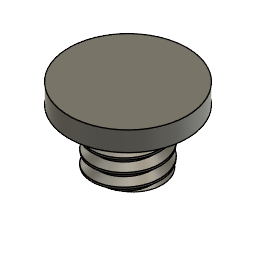
M2.5 x 6mm Phillips Flat Head Screw (Autodesk Fusion 360 design; units mm, degrees)
part number: 2026-08-01-20-11-09-453
Autodesk Fusion 360 part; units mm, degrees
sketch "Sketch1" plane through (0, 0, 0) normal (0, 1, 0) x (1, 0, 0)
  circle A0 centre (0, 0) radius 1.5
  dimension "d1" = 3
  constraint coincident A0.centre origin
  measures "d1" diameter of A0
extrude "Extrude1" add sketch "Sketch1" along normal blind 2
thread "Thread1" "ISO Metric profile 2.5 M2.5x0.45 M2.5x0.45 6g" major diameter 2.43 minor diameter 1.9165 pitch 0.45 angle 60 modelled right hand crest width 0.0648 on face at (1.4981, 1.3333, 0.0748) crest through (1.215, -0.1125, 0)
sketch "Sketch2" plane through (0, 2, 0) normal (0, 1, 0) x (-1, 0, 0)
  spline S0 degree 3 poles (-0.1252, 1.2085) (-0.2764, 1.1771) (-0.4201, 1.117) (-0.6707, 0.9476) (-0.7764, 0.8419) (-0.9369, 0.6004) (-0.9921, 0.4683) (-1.0464, 0.1962) (-1.0473, 0.0593) (-1.0042, -0.1619) (-0.9753, -0.2474) (-0.8966, -0.4057) (-0.8477, -0.4781) (-0.7897, -0.5428) knots 0 0 0 0 0.046326 0.046326 0.090815 0.090815 0.133466 0.133466 0.17428 0.17428 0.201332 0.201332 0.227524 0.227524 0.227524 0.227524
  arc A0 (-0.7897, -0.5428) -> (0.2561, -0.9234) centre (0, 0) ccw
  spline S1 degree 3 poles (0.2561, -0.9234) (0.3815, -0.9055) (0.5022, -0.8627) (0.7262, -0.7312) (0.8263, -0.6416) (0.9913, -0.4249) (1.0527, -0.2985) (1.1264, -0.0233) (1.1356, 0.1233) (1.1038, 0.3714) (1.0763, 0.4727) (0.9942, 0.6681) (0.9393, 0.7609) (0.8727, 0.8453) knots 0 0 0 0 0.038021 0.038021 0.077873 0.077873 0.119555 0.119555 0.163068 0.163068 0.19429 0.19429 0.22638 0.22638 0.22638 0.22638
  arc A1 (0.8727, 0.8453) -> (-0.1252, 1.2085) centre (0, 0) ccw
  circle A2 centre (0, 0) radius 2.1
  dimension "d6" = 4.2
  constraint coincident A0.centre A1.centre
  measures "d6" diameter of A2
extrude "Extrude2" add sketch "Sketch2" along normal blind 0.7 contours S0 A0 S1 A1 | A2
